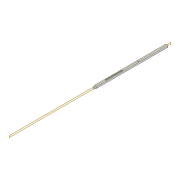
# Autodesk Inventor part: Part_8
Saved by Autodesk Inventor 2022 (Build 260153000, 153)
## iProperties
Created: 2022-05-03
Part Number: Part_8
Material: Generic
Document SubType Name: Modeling
Designer: dell
Density: 1 g/cm^3
Appearance: Default
Author: dell
Autodesk Inventor part; units mm, degrees
ref_plane "XZ Plane" through (0, 0, 0) normal (0, 1, 0) x (-1, 0, 0)
ref_plane "XY Plane" through (0, 0, 0) normal (0, 0, 1) x (1, 0, 0)
sketch "Sketch1" plane through (0, 0, 0) normal (0, 1, 0) x (-1, 0, 0)
  line L0 (0, 0) -> (0, -405.743) construction
  line L1 (-4, 0) -> (-4, -405.743)
  line L2 (4, -405.743) -> (4, 0)
  arc A0 (4, 0) -> (-4, 0) centre (0, 0) ccw
  arc A1 (-4, -405.743) -> (4, -405.743) centre (0, -405.743) ccw
  circle A2 centre (0, 0) radius 1.5
  circle A3 centre (0, -405.743) radius 1.5
  line L3 (0, -347.063) -> (0, -288.743) construction
  line L4 (1.5, -347.063) -> (1.5, -288.743)
  line L5 (-1.5, -288.743) -> (-1.5, -347.063)
  arc A4 (-1.5, -347.063) -> (1.5, -347.063) centre (0, -347.063) ccw
  arc A5 (1.5, -288.743) -> (-1.5, -288.743) centre (0, -288.743) ccw
  line L6 (0, -405.743) -> (0, -505.743) construction
  line L7 (-4, -405.743) -> (-4, -505.743)
  line L8 (4, -505.743) -> (4, -405.743)
  arc A6 (4, -405.743) -> (-4, -405.743) centre (0, -405.743) ccw
  arc A7 (-4, -505.743) -> (4, -505.743) centre (0, -505.743) ccw
  point P0 (0, -202.8715)
  point P1 (0, -317.903)
  point P2 (0, -455.743)
  dimension "d0" = 8
  dimension "d1" = 405.743
  dimension "d2" = 3
  dimension "d3" = 3
  dimension "d20" = 3
  dimension "d21" = 58.68
  dimension "d22" = 117
  dimension "d23" = 8
  dimension "d24" = 100
  constraints: 24 end point, 12 point on circle, 12 tangent, 8 centre point, 3 midpoint, 3 parallel, 3 point on line, 2 coincident, 1 vertical
  measures "d0" diameter of A1
  measures "d1" distance of L0.end L0.start
  measures "d2" diameter of A2
  measures "d3" diameter of A3
  measures "d20" diameter of A5
  measures "d21" distance of L0.end L3.start
  measures "d22" distance of L0.end L3.end
  measures "d23" diameter of A7
  measures "d24" distance of L0.end L6.end
extrude "Extrusion1" add sketch "Sketch1" along normal blind 6
sketch "Sketch2" plane through (0, 6, 0) normal (0, 1, 0) x (1, 0, 0)
  line L0 (-4, 505.743) -> (-4, 0) projected
  arc A0 (-4, 0) -> (4, 0) centre (0, 0) ccw projected
  line L1 (4, 0) -> (4, 505.743) projected
  arc A1 (4, 505.743) -> (-4, 505.743) centre (0, 505.743) ccw projected
  arc A2 (1.5, 347.063) -> (-1.5, 347.063) centre (0, 347.063) ccw projected
  line L2 (1.5, 347.063) -> (1.5, 288.743) projected
  arc A3 (-1.5, 288.743) -> (1.5, 288.743) centre (0, 288.743) ccw projected
  line L3 (-1.5, 288.743) -> (-1.5, 347.063) projected
  circle A4 centre (0, 405.743) radius 1.5 projected
  circle A5 centre (0, 0) radius 1.5 projected
  line L4 (-4, 505.743) -> (-4, 0) projected
  line L5 (-4, 252.8715) -> (0, 244.2935)
  line L6 (0, 244.2935) -> (4, 252.8715)
  line L7 (4, 0) -> (4, 505.743) projected
  dimension "d25" = 25
  dimension "d26" = 25
  constraints: 4 end point, 2 midpoint
  measures "d25" angle of L0 L5
  measures "d26" angle of L1 L6
extrude "Extrusion2" cut sketch "Sketch2" against normal blind 10 contours L5 L6 L1 A0 L0
body "Solid1"
